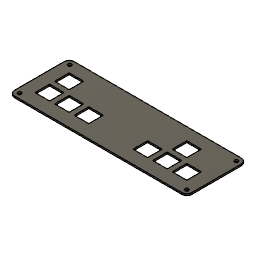
Celeste Hackpad Top (Autodesk Fusion 360 design; units mm, degrees)
part number: 2025-12-01-19-37-04-228
Autodesk Fusion 360 part; units mm, degrees
sketch "plate" plane through (0, 0, 0) normal (0, 0, 1) x (1, 0, 0)
  line L0 (3.025, -2.525) -> (16.025, -2.525)
  line L1 (3.025, -16.525) -> (16.025, -16.525)
  line L2 (2.525, -3.025) -> (2.525, -16.025)
  line L3 (16.525, -3.025) -> (16.525, -16.025)
  arc A0 (3.025, -2.525) -> (2.525, -3.025) centre (3.025, -3.025) ccw
  arc A1 (16.525, -3.025) -> (16.025, -2.525) centre (16.025, -3.025) ccw
  arc A2 (2.525, -16.025) -> (3.025, -16.525) centre (3.025, -16.025) ccw
  arc A3 (16.025, -16.525) -> (16.525, -16.025) centre (16.025, -16.025) ccw
  line L4 (117.325, -2.525) -> (130.325, -2.525)
  line L5 (117.325, -16.525) -> (130.325, -16.525)
  line L6 (116.825, -3.025) -> (116.825, -16.025)
  line L7 (130.825, -3.025) -> (130.825, -16.025)
  arc A4 (117.325, -2.525) -> (116.825, -3.025) centre (117.325, -3.025) ccw
  arc A5 (130.825, -3.025) -> (130.325, -2.525) centre (130.325, -3.025) ccw
  arc A6 (116.825, -16.025) -> (117.325, -16.525) centre (117.325, -16.025) ccw
  arc A7 (130.325, -16.525) -> (130.825, -16.025) centre (130.325, -16.025) ccw
  line L8 (3.025, -21.575) -> (16.025, -21.575)
  line L9 (3.025, -35.575) -> (16.025, -35.575)
  line L10 (2.525, -22.075) -> (2.525, -35.075)
  line L11 (16.525, -22.075) -> (16.525, -35.075)
  arc A8 (3.025, -21.575) -> (2.525, -22.075) centre (3.025, -22.075) ccw
  arc A9 (16.525, -22.075) -> (16.025, -21.575) centre (16.025, -22.075) ccw
  arc A10 (2.525, -35.075) -> (3.025, -35.575) centre (3.025, -35.075) ccw
  arc A11 (16.025, -35.575) -> (16.525, -35.075) centre (16.025, -35.075) ccw
  line L12 (22.075, -21.575) -> (35.075, -21.575)
  line L13 (22.075, -35.575) -> (35.075, -35.575)
  line L14 (21.575, -22.075) -> (21.575, -35.075)
  line L15 (35.575, -22.075) -> (35.575, -35.075)
  arc A12 (22.075, -21.575) -> (21.575, -22.075) centre (22.075, -22.075) ccw
  arc A13 (35.575, -22.075) -> (35.075, -21.575) centre (35.075, -22.075) ccw
  arc A14 (21.575, -35.075) -> (22.075, -35.575) centre (22.075, -35.075) ccw
  arc A15 (35.075, -35.575) -> (35.575, -35.075) centre (35.075, -35.075) ccw
  line L16 (41.125, -21.575) -> (54.125, -21.575)
  line L17 (41.125, -35.575) -> (54.125, -35.575)
  line L18 (40.625, -22.075) -> (40.625, -35.075)
  line L19 (54.625, -22.075) -> (54.625, -35.075)
  arc A16 (41.125, -21.575) -> (40.625, -22.075) centre (41.125, -22.075) ccw
  arc A17 (54.625, -22.075) -> (54.125, -21.575) centre (54.125, -22.075) ccw
  arc A18 (40.625, -35.075) -> (41.125, -35.575) centre (41.125, -35.075) ccw
  arc A19 (54.125, -35.575) -> (54.625, -35.075) centre (54.125, -35.075) ccw
  line L20 (98.275, -21.575) -> (111.275, -21.575)
  line L21 (98.275, -35.575) -> (111.275, -35.575)
  line L22 (97.775, -22.075) -> (97.775, -35.075)
  line L23 (111.775, -22.075) -> (111.775, -35.075)
  arc A20 (98.275, -21.575) -> (97.775, -22.075) centre (98.275, -22.075) ccw
  arc A21 (111.775, -22.075) -> (111.275, -21.575) centre (111.275, -22.075) ccw
  arc A22 (97.775, -35.075) -> (98.275, -35.575) centre (98.275, -35.075) ccw
  arc A23 (111.275, -35.575) -> (111.775, -35.075) centre (111.275, -35.075) ccw
  line L24 (117.325, -21.575) -> (130.325, -21.575)
  line L25 (117.325, -35.575) -> (130.325, -35.575)
  line L26 (116.825, -22.075) -> (116.825, -35.075)
  line L27 (130.825, -22.075) -> (130.825, -35.075)
  arc A24 (117.325, -21.575) -> (116.825, -22.075) centre (117.325, -22.075) ccw
  arc A25 (130.825, -22.075) -> (130.325, -21.575) centre (130.325, -22.075) ccw
  arc A26 (116.825, -35.075) -> (117.325, -35.575) centre (117.325, -35.075) ccw
  arc A27 (130.325, -35.575) -> (130.825, -35.075) centre (130.325, -35.075) ccw
  line L28 (136.375, -21.575) -> (149.375, -21.575)
  line L29 (136.375, -35.575) -> (149.375, -35.575)
  line L30 (135.875, -22.075) -> (135.875, -35.075)
  line L31 (149.875, -22.075) -> (149.875, -35.075)
  arc A28 (136.375, -21.575) -> (135.875, -22.075) centre (136.375, -22.075) ccw
  arc A29 (149.875, -22.075) -> (149.375, -21.575) centre (149.375, -22.075) ccw
  arc A30 (135.875, -35.075) -> (136.375, -35.575) centre (136.375, -35.075) ccw
  arc A31 (149.375, -35.575) -> (149.875, -35.075) centre (149.375, -35.075) ccw
  line L32 (-9.515, 9.515) -> (162.885, 9.515)
  line L33 (162.885, 9.515) -> (162.885, -48.585)
  line L34 (162.885, -48.585) -> (-9.515, -48.585)
  line L35 (-9.515, -48.585) -> (-9.515, 9.515)
  circle A32 centre (-4, 4.515) radius 1.7
  circle A33 centre (157.885, 4.515) radius 1.7
  circle A34 centre (157.885, -43.585) radius 1.7
  circle A35 centre (-4.515, -43.585) radius 1.7
  dimension "d1" = 172.4
  dimension "d2" = 58.1
  dimension "d3" = 12.04
  dimension "d4" = 12.04
  dimension "d5" = 3.4
  dimension "d6" = 5
  dimension "d7" = 5.515
  dimension "d8" = 3.4
  dimension "d9" = 5
  dimension "d10" = 5
  dimension "d11" = 3.4
  dimension "d12" = 5
  dimension "d13" = 5
  dimension "d14" = 3.4
  dimension "d15" = 5
  dimension "d16" = 5
  constraint horizontal L32
  constraint vertical L33
  constraint horizontal L34
  constraint vertical L35
  measures "d1" distance of L32.start L32.end
  measures "d2" distance of L32.start L34.end
  measures "d3" distance of L0 L32
  measures "d4" distance of L2 L35
  measures "d5" diameter of A32
  measures "d6" distance of L32 A32.centre
  measures "d7" distance of L35 A32.centre
  measures "d8" diameter of A33
  measures "d9" distance of L33 A33.centre
  measures "d10" distance of L32 A33.centre
  measures "d11" diameter of A34
  measures "d12" distance of L33 A34.centre
  measures "d13" distance of L34 A34.centre
  measures "d14" diameter of A35
  measures "d15" distance of L34 A35.centre
  measures "d16" distance of L35 A35.centre
extrude "Extrude1" add sketch "plate" along normal blind 1.5
fillet "Fillet1" radius 5 4 edges at (162.885, -48.585, 0.75) (162.885, 9.515, 0.75) (-9.515, 9.515, 0.75) (-9.515, -48.585, 0.75)
